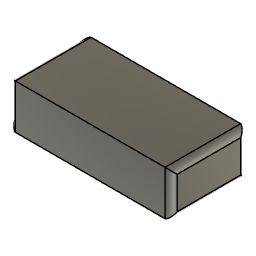
Curtain Connector Simple (Autodesk Fusion 360 design; units mm, degrees)
Autodesk Fusion 360 part; units mm, degrees
sketch "Sketch1" plane through (0, 0, 0) normal (0, 0, 1) x (1, 0, 0)
  line L0 (0, 0) -> (40, 0)
  line L1 (40, 0) -> (40, 18.7)
  line L2 (40, 18.7) -> (0, 18.7)
  line L3 (0, 18.7) -> (0, 0)
  dimension "d1" = 18.7
  constraint horizontal L0
  constraint vertical L1
  constraint horizontal L2
  constraint vertical L3
  constraint coincident L0.start L3.end
  measures "d1" distance of L0.end L1.end
extrude "Extrude1" add sketch "Sketch1" along normal blind 11
fillet "Fillet1" radius 1.5 tangency weight 0.4303 2 faces at (40, 6.2333, 7.3333) (0, 12.4667, 7.3333)
